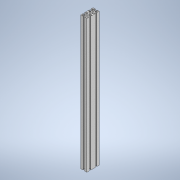
# Autodesk Inventor part: Part2
Saved by Autodesk Inventor 2022 (Build 260153000, 153)
## iProperties
Created: 2021-10-05
Part Number: Part2
Material: Generic
Document SubType Name: Modeling
Designer: Administrator
Density: 1 g/cm^3
Appearance: Aluminum Cast
Mass: 467.574 g
Surface Area: 4247.19 cm^2
Volume: 467.574 cm^3
Author: Administrator
Autodesk Inventor part; units mm, degrees
ref_plane "YZ Plane" through (0, 0, 0) normal (1, 0, 0) x (0, 1, 0)
ref_plane "XY Plane" through (0, 0, 0) normal (0, 0, 1) x (1, 0, 0)
ref_plane "Work Plane1" through (0, 431, 0) normal (0, 1, 0) x (-1, 0, 0)
sketch "Sketch1" plane through (0, 431, 0) normal (0, 1, 0) x (-1, 0, 0)
  line L0 (-54.5291, -19.1661) -> (-51.4685, -22.2268)
  line L1 (-67.4685, 2.2039) -> (-67.4685, -12.5361)
  line L2 (-51.4685, 11.8946) -> (-54.5291, 8.8339)
  line L3 (-48.9685, -9.1661) -> (-48.9685, -12.5361)
  line L4 (-64.5291, -1.1661) -> (-65.9685, -1.1661)
  line L5 (-54.8385, 14.8339) -> (-54.8385, 13.3339)
  line L6 (-63.4685, -23.6661) -> (-63.4685, -22.2268)
  line L7 (-53.4685, -18.1054) -> (-53.4685, -12.2268)
  line L8 (-67.4685, -25.1661) -> (-60.0985, -25.1661)
  line L9 (-48.9685, 7.4639) -> (-47.4685, 7.4639)
  line L10 (-63.4685, -2.2268) -> (-60.4078, 0.8339)
  line L11 (-48.9685, -17.7961) -> (-48.9685, -21.1661)
  line L12 (-64.5291, 10.8339) -> (-61.4685, 7.7732)
  line L13 (-53.4685, 7.7732) -> (-50.4078, 10.8339)
  line L14 (-54.5291, -11.1661) -> (-60.4078, -11.1661)
  line L15 (-65.9685, -21.1661) -> (-65.9685, -17.7961)
  line L16 (-67.4685, 7.4639) -> (-65.9685, 7.4639)
  line L17 (-60.0985, 13.3339) -> (-60.0985, 14.8339)
  line L18 (-61.4685, -12.2268) -> (-61.4685, -18.1054)
  line L19 (-47.4685, -25.1661) -> (-47.4685, -17.7961)
  line L20 (-48.9685, -1.1661) -> (-50.4078, -1.1661)
  line L21 (-47.4685, -12.5361) -> (-47.4685, 2.2039)
  line L22 (-51.4685, -23.6661) -> (-54.8385, -23.6661)
  line L23 (-65.9685, -12.5361) -> (-65.9685, -9.1661)
  line L24 (-60.4078, 8.8339) -> (-63.4685, 11.8946)
  line L25 (-50.4078, -9.1661) -> (-48.9685, -9.1661)
  line L26 (-51.4685, 13.3339) -> (-51.4685, 11.8946)
  line L27 (-60.4078, -19.1661) -> (-54.5291, -19.1661)
  line L28 (-65.9685, 2.2039) -> (-67.4685, 2.2039)
  line L29 (-50.4078, -21.1661) -> (-53.4685, -18.1054)
  line L30 (-47.4685, 14.8339) -> (-54.8385, 14.8339)
  line L31 (-61.4685, 1.8946) -> (-64.5291, -1.1661)
  line L32 (-54.5291, 0.8339) -> (-51.4685, -2.2268)
  line L33 (-60.0985, -23.6661) -> (-63.4685, -23.6661)
  line L34 (-67.4685, -17.7961) -> (-67.4685, -25.1661)
  line L35 (-65.9685, 10.8339) -> (-64.5291, 10.8339)
  line L36 (-47.4685, -17.7961) -> (-48.9685, -17.7961)
  line L37 (-48.9685, 10.8339) -> (-48.9685, 7.4639)
  line L38 (-63.4685, -8.1054) -> (-63.4685, -2.2268)
  line L39 (-53.4685, 1.8946) -> (-53.4685, 7.7732)
  line L40 (-51.4685, -8.1054) -> (-54.5291, -11.1661)
  line L41 (-67.4685, 14.8339) -> (-67.4685, 7.4639)
  line L42 (-64.5291, -21.1661) -> (-65.9685, -21.1661)
  line L43 (-54.8385, -25.1661) -> (-47.4685, -25.1661)
  line L44 (-63.4685, 13.3339) -> (-60.0985, 13.3339)
  line L45 (-48.9685, 2.2039) -> (-48.9685, -1.1661)
  line L46 (-64.5291, -9.1661) -> (-61.4685, -12.2268)
  line L47 (-51.4685, -22.2268) -> (-51.4685, -23.6661)
  line L48 (-48.9685, -12.5361) -> (-47.4685, -12.5361)
  line L49 (-67.4685, -12.5361) -> (-65.9685, -12.5361)
  line L50 (-54.5291, 8.8339) -> (-60.4078, 8.8339)
  line L51 (-65.9685, -1.1661) -> (-65.9685, 2.2039)
  line L52 (-53.4685, -12.2268) -> (-50.4078, -9.1661)
  line L53 (-54.8385, 13.3339) -> (-51.4685, 13.3339)
  line L54 (-63.4685, -22.2268) -> (-60.4078, -19.1661)
  line L55 (-47.4685, 7.4639) -> (-47.4685, 14.8339)
  line L56 (-60.4078, 0.8339) -> (-54.5291, 0.8339)
  line L57 (-48.9685, -21.1661) -> (-50.4078, -21.1661)
  line L58 (-61.4685, 7.7732) -> (-61.4685, 1.8946)
  line L59 (-60.0985, -25.1661) -> (-60.0985, -23.6661)
  line L60 (-60.4078, -11.1661) -> (-63.4685, -8.1054)
  line L61 (-65.9685, 7.4639) -> (-65.9685, 10.8339)
  line L62 (-50.4078, 10.8339) -> (-48.9685, 10.8339)
  line L63 (-65.9685, -17.7961) -> (-67.4685, -17.7961)
  line L64 (-50.4078, -1.1661) -> (-53.4685, 1.8946)
  line L65 (-61.4685, -18.1054) -> (-64.5291, -21.1661)
  line L66 (-51.4685, -2.2268) -> (-51.4685, -8.1054)
  line L67 (-60.0985, 14.8339) -> (-67.4685, 14.8339)
  line L68 (-54.8385, -23.6661) -> (-54.8385, -25.1661)
  line L69 (-63.4685, 11.8946) -> (-63.4685, 13.3339)
  line L70 (-65.9685, -9.1661) -> (-64.5291, -9.1661)
  line L71 (-47.4685, 2.2039) -> (-48.9685, 2.2039)
  constraints: 144 end point, 61 equal length, 28 horizontal, 28 vertical, 19 collinear, 3 perpendicular, 1 parallel
extrude "Extrusion1" add sketch "Sketch1" against normal blind 431
hole "Hole2" at (57.4685, 431, 4.8339) direction (0, -1, 0) diameter 4 depth 431 tip angle 118
sketch "Sketch2" plane through (0, 431, 0) normal (0, 1, 0) x (-1, 0, 0)
  point P0 (-57.4685, 4.8339)
hole "Hole1" at (57.4685, 431, -15.1661) direction (0, -1, 0) diameter 4 depth 431 tip angle 118
sketch "Sketch3" plane through (0, 431, 0) normal (0, 1, 0) x (-1, 0, 0)
  point P0 (-57.4685, -15.1661)
body "Solid3"
